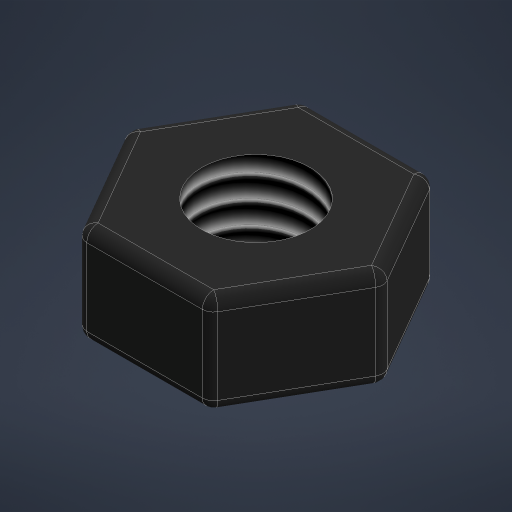
# Autodesk Inventor part: M2 Nut
Saved by Autodesk Inventor 2024 (Build 280153000, 153)
## iProperties
Created: 2024-10-26
Part Number: M2 Nut
Material: Generic
Document SubType Name: Modeling
Designer: jerem
Density: 1 g/cm^3
Appearance: Default
Author: jerem
Autodesk Inventor part; units mm, degrees
ref_plane "YZ Plane" through (0, 0, 0) normal (1, 0, 0) x (0, 1, 0)
ref_plane "XZ Plane" through (0, 0, 0) normal (0, 1, 0) x (-1, 0, 0)
ref_plane "XY Plane" through (0, 0, 0) normal (0, 0, 1) x (1, 0, 0)
sketch "Sketch1" plane through (0, 0, 0) normal (0, 1, 0) x (-1, 0, 0)
  line L0 (2.2632, 0) -> (1.1316, -1.96)
  line L1 (1.1316, -1.96) -> (-1.1316, -1.96)
  line L2 (-1.1316, -1.96) -> (-2.2632, 0)
  line L3 (-2.2632, 0) -> (-1.1316, 1.96)
  line L4 (-1.1316, 1.96) -> (1.1316, 1.96)
  line L5 (1.1316, 1.96) -> (2.2632, 0)
  circle A0 centre (0, 0) radius 0.95
  dimension "d0" = 3.92
  dimension "d1" = 1.9
  constraints: 12 end point, 2 coincident, 1 centre point, 1 horizontal, 13 other
  measures "d0" distance between parallel lines of L4 L1
  measures "d1" diameter of A0
extrude "Extrusion1" add sketch "Sketch1" along normal blind 1.75
fillet "Fillet1" radius 0.2 18 edges at (1.6974, 1.75, 0.98) (0, 1.75, 1.96) (1.1316, 0.875, 1.96) (0, 0, 1.96) (-1.1316, 0.875, 1.96) (1.6974, 0, 0.98) (2.2632, 0.875, 0) (1.1316, 0.875, -1.96) (1.6974, 1.75, -0.98) (1.6974, 0, -0.98) (-1.1316, 0.875, -1.96) (0, 1.75, -1.96) (0, 0, -1.96) (-1.6974, 1.75, 0.98) (-1.6974, 1.75, -0.98) (-2.2632, 0.875, 0) (-1.6974, 0, -0.98) (-1.6974, 0, 0.98)
thread "Thread1" size "M2x0.4" class "6H" standard "ANSI Metric M Profile" full length
body "Solid1"
